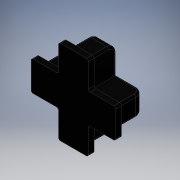
# Autodesk Inventor part: Cross
Saved by Autodesk Inventor 2016 SP1 (Build 200210100, 210)
## iProperties
Created: 2018-06-05
Part Number: Cross
Material: Plastique ABS
Document SubType Name: Modeling
Designer: dimercur
Density: 1.06 g/cm^3
Appearance: Lisse - Noir
Author: dimercur
Autodesk Inventor part; units mm, degrees
ref_plane "YZ Plane" through (0, 0, 0) normal (1, 0, 0) x (0, 1, 0)
ref_plane "XZ Plane" through (0, 0, 0) normal (0, 1, 0) x (-1, 0, 0)
ref_plane "XY Plane" through (0, 0, 0) normal (0, 0, 1) x (1, 0, 0)
sketch "Esquisse1" plane through (0, 0, 0) normal (0, 1, 0) x (-1, 0, 0)
  line L0 (9.5, 2.5) -> (-9.5, 2.5)
  line L1 (-9.5, 2.5) -> (-9.5, -2.5)
  line L2 (-9.5, -2.5) -> (9.5, -2.5)
  line L3 (9.5, -2.5) -> (9.5, 2.5)
  line L4 (2.5, 9.5) -> (-2.5, 9.5)
  line L5 (-2.5, 9.5) -> (-2.5, -9.5)
  line L6 (-2.5, -9.5) -> (2.5, -9.5)
  line L7 (2.5, -9.5) -> (2.5, 9.5)
  point P0 (0, 0)
  dimension "d0" = 19
  dimension "d1" = 19
  dimension "d2" = 5
  dimension "d3" = 5
  dimension "d4" = 7
  dimension "d5" = 7
  dimension "d6" = 2.5
  dimension "d7" = 2.5
  constraints: 16 end point, 4 parallel, 2 horizontal, 2 perpendicular
  measures "d0" distance of L0.start L0.end
  measures "d1" distance of L6.end L4.start
  measures "d2" distance of L4.start L4.end
  measures "d3" distance of L2.end L0.start
  measures "d4" distance from line of L0 L4.start
  measures "d5" distance from line of L7 L0.start
  measures "d6" vertical distance of point (0, 0) L0.start
  measures "d7" horizontal distance of point (0, 0) L4.start
extrude "Extrusion1" add sketch "Esquisse1" along normal blind 7
sketch "Esquisse2" plane through (0, 0, 0) normal (0, -1, 0) x (1, 0, 0)
  line L0 (2.5, 9.5) -> (2.5, 2.5) projected
  line L1 (-2.5, 9.5) -> (2.5, 9.5) projected
  line L2 (-2.5, 2.5) -> (-2.5, 9.5) projected
  line L3 (-9.5, 2.5) -> (-2.5, 2.5) projected
  line L4 (-9.5, -2.5) -> (-9.5, 2.5) projected
  line L5 (-2.5, -2.5) -> (-9.5, -2.5) projected
  line L6 (-2.5, -9.5) -> (-2.5, -2.5) projected
  line L7 (2.5, -9.5) -> (-2.5, -9.5) projected
  line L8 (2.5, -2.5) -> (2.5, -9.5) projected
  line L9 (9.5, -2.5) -> (2.5, -2.5) projected
  line L10 (9.5, 2.5) -> (9.5, -2.5) projected
  line L11 (2.5, 2.5) -> (9.5, 2.5) projected
  line L12 (10.8, 3.8) -> (10.8, -3.8)
  line L13 (10.8, -3.8) -> (3.8, -3.8)
  line L14 (3.8, -3.8) -> (3.8, -10.8)
  line L15 (3.8, -10.8) -> (-3.8, -10.8)
  line L16 (-3.8, -10.8) -> (-3.8, -3.8)
  line L17 (-3.8, -3.8) -> (-10.8, -3.8)
  line L18 (-10.8, -3.8) -> (-10.8, 3.8)
  line L19 (-10.8, 3.8) -> (-3.8, 3.8)
  line L20 (-3.8, 3.8) -> (-3.8, 10.8)
  line L21 (-3.8, 10.8) -> (3.8, 10.8)
  line L22 (3.8, 10.8) -> (3.8, 3.8)
  line L23 (3.8, 3.8) -> (10.8, 3.8)
  point P0 (0, 0)
  dimension "d10" = 1.3
  constraints: 24 end point, 11 other
  measures "d10" distance between parallel lines of L0 L22
extrude "Extrusion2" add sketch "Esquisse2" along normal blind 1.5 contours L0 L11 L10 L9 L8 L7 L6 L5 L4 L3 L2 L1 | L12 L13 L14 L15 L16 L17 L18 L19 L20 L21 L22 L23
fillet "Congé1" radius 2 4 edges at (0, 7, 9.5) (9.5, 7, 0) (0, 7, -9.5) (-9.5, 7, 0)
fillet "Congé2" radius 0.5 24 edges at (2.5, 6.4142, 8.9142) (2.5, 2.5, 9.5) (2.5, 7, 5) (8.9142, 6.4142, 2.5) (9.5, 2.5, 2.5) (5, 7, 2.5) (8.9142, 6.4142, -2.5) (9.5, 2.5, -2.5) (5, 7, -2.5) (2.5, 6.4142, -8.9142) (2.5, 2.5, -9.5) (2.5, 7, -5) (-2.5, 6.4142, -8.9142) (-2.5, 2.5, -9.5) (-2.5, 7, -5) (-8.9142, 6.4142, -2.5) (-9.5, 2.5, -2.5) (-5, 7, -2.5) (-8.9142, 6.4142, 2.5) (-9.5, 2.5, 2.5) (-5, 7, 2.5) (-2.5, 6.4142, 8.9142) (-2.5, 2.5, 9.5) (-2.5, 7, 5)
fillet "Congé3" radius 0.5 12 edges at (10.8, -0.75, -3.8) (10.8, -0.75, 3.8) (3.8, -0.75, -3.8) (3.8, -0.75, -10.8) (-3.8, -0.75, -10.8) (-3.8, -0.75, -3.8) (-10.8, -0.75, -3.8) (-10.8, -0.75, 3.8) (-3.8, -0.75, 3.8) (-3.8, -0.75, 10.8) (3.8, -0.75, 10.8) (3.8, -0.75, 3.8)
sketch "Esquisse3" plane through (0, 7, 0) normal (0, 1, 0) x (1, 0, 0)
  line L0 (1.1, -4.5) -> (-1.2682, -4.5)
  line L1 (-1.2682, -4.5) -> (0, -6.5)
  line L2 (1.1, -4.5) -> (0, -6.5)
  line L3 (2.5, -7.5) -> (2.5, -2.5) projected
  line L4 (-2, -9.5) -> (2, -9.5) projected
  line L5 (-4.5, -1.1) -> (-4.5, 1.2682)
  line L6 (-4.5, 1.2682) -> (-6.5, 0)
  line L7 (-4.5, -1.1) -> (-6.5, 0)
  line L8 (-1.1, 4.5) -> (1.2682, 4.5)
  line L9 (1.2682, 4.5) -> (0, 6.5)
  line L10 (-1.1, 4.5) -> (0, 6.5)
  line L11 (4.5, 1.1) -> (4.5, -1.2682)
  line L12 (4.5, -1.2682) -> (6.5, 0)
  line L13 (4.5, 1.1) -> (6.5, 0)
  point P0 (0, 0)
  point P1 (0, 0)
  point P2 (0, 0)
  point P3 (0, 0)
  dimension "d18" = 1.1
  dimension "d19" = 2.5
  dimension "d20" = 3
  dimension "d21" = 5
  dimension "d24" = 360
  constraints: 24 end point, 2 coincident, 1 equal length, 1 horizontal, 26 other
  measures "d18" horizontal distance of point (0, 0) L0.start
  measures "d19" distance from line of L3 L1.end
  measures "d20" distance from line of L4 L1.end
  measures "d21" distance between parallel lines of L4 L0
extrude "Extrusion3" cut sketch "Esquisse3" against normal blind 0.2
equation "\"d1\" = d0"
equation "\"d3\" = d2"
equation "\"d4\" = -0.5 * d2 + 0.5 * d0"
equation "\"d5\" = d4"
equation "\"d6\" = 0.5 * d3"
equation "\"d7\" = 0.5 * d2"
equation "\"d18\" = 0.5 * d17"
equation "\"d17\" = 2.2"
